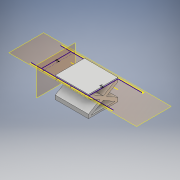
# Autodesk Inventor part: legspacer_paula
Saved by Autodesk Inventor 2018 (Build 220112000, 112)
## iProperties
Created: 2019-11-13
Part Number: legspacer_paula
Material: Generic
Document SubType Name: Modeling
Designer: bitbots
Density: 1 g/cm^3
Appearance: Default
Author: bitbots
Autodesk Inventor part; units mm, degrees
ref_plane "YZ Plane" through (0, 0, 0) normal (1, 0, 0) x (0, 1, 0)
ref_plane "XZ Plane" through (0, 0, 0) normal (0, 1, 0) x (-1, 0, 0)
ref_plane "XY Plane" through (0, 0, 0) normal (0, 0, 1) x (1, 0, 0)
ref_plane "Work Plane1" through (32.4858, 0, 0) normal (0, 0, 1) x (1, 0, 0)
sketch "Sketch1" plane through (32.4858, 0, 0) normal (0, 0, 1) x (1, 0, 0)
  line L0 (-82.3611, -0.4) -> (-82.3611, 2.4)
  line L1 (-32.4858, 2) -> (-181.2976, 2)
  line L2 (-32.4858, 55) -> (-181.2976, 55)
  line L3 (-82.3611, 54.6) -> (-82.3611, 57.4)
  line L4 (-157.3611, 54.6) -> (-157.3611, 57.4)
  line L5 (-157.3611, -0.4) -> (-157.3611, 2.4)
  line L6 (-107.3611, -0.4) -> (-107.3611, 2.4)
  line L7 (-132.3611, -0.4) -> (-132.3611, 2.4)
  line L8 (-107.3611, 54.6) -> (-107.3611, 57.4)
  line L9 (-132.3611, 54.6) -> (-132.3611, 57.4)
  line L10 (-32.4858, 0) -> (-181.2976, 0) projected
  line L11 (-32.4858, 57) -> (-181.2976, 57) projected
  line L12 (-82.3611, 2) -> (-82.3611, 55) construction
  line L13 (-157.3611, 2) -> (-157.3611, 55) construction
  line L14 (-77.3611, 2) -> (-77.3611, 55)
  line L15 (-162.3611, 2) -> (-162.3611, 55)
  dimension "d0" = 5
  dimension "d1" = 5
  constraints: 28 end point, 8 point on line, 8 vertical, 2 horizontal, 2 parallel, 20 other
  measures "d0" distance between parallel lines of L12 L14
  measures "d1" distance between parallel lines of L13 L15
ref_plane "Work Plane3" through (-129.8754, 2, 0) normal (1, 0, 0) x (0, 1, 0)
ref_plane "Work Plane2" through (1.0604, 0, 0) normal (0, 0, 1) x (-1, 0, 0)
sketch "Sketch2" plane through (-129.8754, 2, 0) normal (1, 0, 0) x (0, 1, 0)
  line L0 (0, 8.3309) -> (0, -17.2762) projected
  line L1 (53, 8.3309) -> (53, -17.2762) projected
  line L2 (53, -34) -> (55, -34) projected
  line L3 (53, -34) -> (55, -34) projected
  line L4 (-2, -34) -> (0, -34) projected
  line L5 (-2, -34) -> (0, -34) projected
  line L6 (53, -34) -> (0, -34) construction
  line L7 (53, -36) -> (0, -36)
  line L8 (0, 0) -> (53, 0) construction
  line L9 (0, 0) -> (0, -8) construction
  line L10 (53, 0) -> (53, -8) construction
  line L11 (47.871, -33) -> (5.129, -33)
  line L12 (53, -29) -> (0, -29) construction
  line L13 (53, 2) -> (0, 2)
  line L14 (47.871, -1) -> (5.129, -1)
  line L15 (53, -5) -> (0, -5) construction
  line L16 (5.129, -33) -> (26.5, -20.5)
  line L17 (32.4839, -17) -> (53, -5)
  line L18 (5.129, -1) -> (26.5, -13.5)
  line L19 (32.4839, -17) -> (53, -29)
  line L20 (0, -29) -> (20.5161, -17)
  line L21 (26.5, -13.5) -> (47.871, -1)
  line L22 (0, -5) -> (20.5161, -17)
  line L23 (26.5, -20.5) -> (47.871, -33)
  line L24 (53, 2) -> (53, -5)
  line L25 (0, 2) -> (0, -5)
  line L26 (0, -29) -> (0, -36)
  line L27 (53, -29) -> (53, -36)
  point P0 (-2, 0)
  dimension "d20" = 2
  dimension "d37" = 1
  dimension "d38" = 4
  dimension "d39" = 2
  dimension "d40" = 1
  dimension "d41" = 4
  constraints: 44 end point, 9 parallel, 4 point on line, 2 collinear, 1 horizontal, 1 vertical
  measures "d20" distance between parallel lines of L6 L7
  measures "d37" distance between parallel lines of L6 L11
  measures "d38" distance between parallel lines of L11 L12
  measures "d39" distance between parallel lines of L8 L13
  measures "d40" distance between parallel lines of L8 L14
  measures "d41" distance between parallel lines of L14 L15
extrude "Extrusion2" add sketch "Sketch2" along normal blind 85
sketch "Sketch3" plane through (-129.8754, 55, -29) normal (0, 1, 0) x (1, 0, 0)
  line L0 (0, -12) -> (85, -12) projected
  point P0 (129.8754, -29)
sketch "Sketch4" plane through (-129.8754, 2, 0) normal (-1, 0, 0) x (0, 0, 1)
  line L0 (-13.5, 26.5) -> (-1, 47.871) projected
  line L1 (-1, 47.871) -> (-1, 5.129) projected
  line L2 (-1, 5.129) -> (-13.5, 26.5) projected
  line L3 (-20.5, 26.5) -> (-33, 5.129) projected
  line L4 (-33, 5.129) -> (-33, 47.871) projected
  line L5 (-33, 47.871) -> (-20.5, 26.5) projected
  line L6 (-36, 53) -> (-36, 0) projected
  line L7 (-36, 0) -> (-29, 0) projected
  line L8 (-29, 0) -> (-17, 20.5161) projected
  line L9 (-17, 20.5161) -> (-5, 0) projected
  line L10 (-5, 0) -> (2, 0) projected
  line L11 (2, 0) -> (2, 53) projected
  line L12 (2, 53) -> (-5, 53) projected
  line L13 (-5, 53) -> (-17, 32.4839) projected
  line L14 (-17, 32.4839) -> (-29, 53) projected
  line L15 (-29, 53) -> (-36, 53) projected
  point P0 (0, -2)
extrude "Extrusion3" cut sketch "Sketch4" against normal blind 25
body "Solid2"
